bart pro xl bed probe bracket (Autodesk Fusion 360 design; units mm, degrees)
Autodesk Fusion 360 part; units mm, degrees
sketch "Sketch1" plane through (0, 0, 0) normal (0, 0, 1) x (1, 0, 0)
  circle A0 centre (25.3818, 25) radius 2
  line L0 (25.3818, 25) -> (25.3777, 25)
  line L1 (25.3777, 25) -> (48.3777, 25) construction
  circle A1 centre (48.3777, 25) radius 2
  line L2 (48.3777, 25) -> (48.3777, 26)
  line L3 (48.3777, 26) -> (48.3777, 32) construction
  line L4 (48.3777, 25) -> (54.3777, 25) construction
  line L5 (54.3777, 25) -> (54.3777, 0) construction
  line L6 (36.8777, 25) -> (36.8777, -5) construction
  line L7 (36.8777, 14.4744) -> (42.8777, 14.4744) construction
  line L8 (36.8777, 14.4744) -> (30.8777, 14.4744) construction
  line L9 (30.8777, 14.4744) -> (30.8777, 25) construction
  line L10 (42.8777, 14.4744) -> (42.8777, 25) construction
  line L11 (42.8777, 14.4744) -> (42.8777, 0) construction
  line L12 (30.8777, 14.4744) -> (30.8777, 0) construction
  line L13 (19.3777, 25) -> (19.3777, 24)
  line L14 (19.3777, 24) -> (19.3777, 0)
  arc A2 (25.3777, 31) -> (19.3777, 25) centre (25.3777, 25) ccw
  arc A3 (54.3777, 25) -> (48.3574, 31) centre (48.3777, 25) ccw
  line L15 (25.3777, 31) -> (48.3574, 31)
  line L16 (54.3777, 25) -> (54.3777, 0)
  line L17 (54.3777, 0) -> (52.8895, 0)
  arc A4 (42.8777, 19.7372) -> (30.8777, 19.7372) centre (36.8777, 18.9484) ccw
  line L18 (30.8777, 19.7372) -> (30.8777, 0)
  line L19 (42.8777, 19.7372) -> (42.8777, 0)
  line L20 (54.3777, 0) -> (42.8777, 0) construction
  line L21 (36.8777, 0) -> (15, 0) construction
  line L22 (19.3777, 0) -> (30.8777, 0)
  line L23 (42.8777, 0) -> (54.3777, 0)
  dimension "d1" = 4
  dimension "d2" = 23
  dimension "d3" = 4
  dimension "d6" = 25
  dimension "d7" = 39.3777
  dimension "d8" = 6
  dimension "d9" = 6
  dimension "d10" = 6
  constraint horizontal L0
  constraint perpendicular L1 L2
  constraint perpendicular L5 L20
  constraint midpoint L1
  constraint perpendicular L6 L20
  constraint coincident L6
  constraint coincident L1
  constraint perpendicular L1 L9
  constraint perpendicular L7 L10
  constraint perpendicular L11 L20
  constraint coincident L20
  constraint perpendicular L12 L20
  constraint perpendicular L14 L20
  constraint tangent A3 L16
  constraint coincident A4
  constraint midpoint L10
  constraint midpoint L9
  constraint perpendicular L18 L22
  constraint perpendicular L19 L22
  constraint collinear L20 L21
  constraint collinear L22 L23
  measures "d1" diameter of A0
  measures "d3" diameter of A1
extrude "Extrude1" add sketch "Sketch1" along normal blind 5
sketch "Sketch2" plane through (0, 0, 0) normal (0, -1, 0) x (1, 0, 0)
  line L0 (19.3777, 0) -> (30.8777, 0)
  line L1 (30.8777, 0) -> (30.8777, 5)
  line L2 (30.8777, 5) -> (19.3777, 5)
  line L3 (19.3777, 5) -> (19.3777, 0)
  line L4 (30.8777, 20) -> (19.3777, 20)
  line L5 (19.3777, 20) -> (19.3777, 0)
  line L6 (30.8777, 0) -> (30.8777, 20)
  dimension "d17" = 20
  constraint horizontal L4
  constraint vertical L5
  constraint perpendicular L4 L6
extrude "Extrude3" add sketch "Sketch2" against normal blind 5 contours L2 L4 L5 L6
sketch "Sketch4" plane through (0, 0, 0) normal (0, -1, 0) x (1, 0, 0)
  line L0 (42.8777, 0) -> (54.3777, 0)
  line L1 (54.3777, 0) -> (54.3777, 5)
  line L2 (54.3777, 5) -> (42.8777, 5)
  line L3 (42.8777, 5) -> (42.8777, 0)
  line L4 (42.8777, 0) -> (42.8777, 20)
  line L5 (54.3777, 0) -> (54.3777, 20)
  line L6 (42.8777, 20) -> (54.3777, 20)
  dimension "d20" = 20
  dimension "d21" = 20
  constraint perpendicular L4 L6
extrude "Extrude4" add sketch "Sketch4" against normal blind 5 contours L2 L4 L5 L6
sketch "Sketch5" plane through (0, 0, 0) normal (0, 1, 0) x (1, 0, 0)
  line L0 (42.8777, -20) -> (54.3777, -20)
  line L1 (37, -20) -> (37, 10) construction
  line L2 (48.3574, -5) -> (25.3777, -5)
  line L3 (42.8777, -5) -> (30.8777, -5)
  line L4 (39.9943, -5) -> (39.9943, -13) construction
  line L5 (39.9943, -13) -> (34, -13) construction
  line L6 (34, -13) -> (34, -19) construction
  circle A0 centre (36.9971, -13) radius 5.95 construction
  dimension "d24" = 8
  dimension "d25" = 6
  dimension "d26" = 11.9
  constraint perpendicular L0 L1
  constraint coincident L2
  constraint perpendicular L1 L5
  constraint midpoint L5
  measures "d26" diameter of A0
sketch "Sketch6" plane through (0, 0, 5) normal (0, 0, 1) x (-1, 0, 0)
  circle A0 centre (-48.3777, -25) radius 2
  circle A1 centre (-25.3818, -25) radius 2
  line L0 (-42.8777, -5) -> (-54.3777, -5)
  line L1 (-54.3777, -5) -> (-54.3777, -25)
  arc A2 (-54.3777, -25) -> (-48.3574, -31) centre (-48.3777, -25) ccw
  line L2 (-48.3574, -31) -> (-25.3777, -31)
  arc A3 (-25.3777, -31) -> (-19.3777, -25) centre (-25.3777, -25) ccw
  line L3 (-19.3777, -25) -> (-19.3777, -5)
  line L4 (-19.3777, -5) -> (-30.8777, -5)
  line L5 (-30.8777, -5) -> (-30.8777, -19.7372)
  arc A4 (-42.8777, -19.7372) -> (-30.8777, -19.7372) centre (-36.8777, -18.9484) ccw
  line L6 (-42.8777, -19.7372) -> (-42.8777, -5)
  line L7 (-28.0277, -26.53) -> (-25.3777, -28.06)
  line L8 (-25.3777, -28.06) -> (-22.7277, -26.53)
  line L9 (-22.7277, -26.53) -> (-22.7277, -23.47)
  line L10 (-22.7277, -23.47) -> (-25.3777, -21.94)
  line L11 (-25.3777, -21.94) -> (-28.0277, -23.47)
  line L12 (-28.0277, -23.47) -> (-28.0277, -26.53)
extrude "Extrude5" cut sketch "Sketch6" against normal blind 2.5 contours L7 L8 L9 L10 L11 L12
sketch "Sketch7" plane through (0, 0, 5) normal (0, 0, 1) x (-1, 0, 0)
  line L0 (-25.3777, -28.06) -> (-28.0277, -26.53)
  line L1 (-28.0277, -26.53) -> (-28.0277, -23.47)
  line L2 (-28.0277, -23.47) -> (-25.3777, -21.94)
  line L3 (-25.3777, -21.94) -> (-22.7277, -23.47)
  line L4 (-22.7277, -23.47) -> (-22.7277, -26.53)
  line L5 (-22.7277, -26.53) -> (-25.3777, -28.06)
  circle A0 centre (-48.3777, -25) radius 2
  line L6 (-42.8777, -5) -> (-54.3777, -5)
  line L7 (-54.3777, -5) -> (-54.3777, -25)
  arc A1 (-54.3777, -25) -> (-48.3574, -31) centre (-48.3777, -25) ccw
  line L8 (-48.3574, -31) -> (-25.3777, -31)
  arc A2 (-25.3777, -31) -> (-19.3777, -25) centre (-25.3777, -25) ccw
  line L9 (-19.3777, -25) -> (-19.3777, -5)
  line L10 (-19.3777, -5) -> (-30.8777, -5)
  line L11 (-30.8777, -5) -> (-30.8777, -19.7372)
  arc A3 (-42.8777, -19.7372) -> (-30.8777, -19.7372) centre (-36.8777, -18.9484) ccw
  line L12 (-42.8777, -19.7372) -> (-42.8777, -5)
  line L13 (-51.0277, -26.53) -> (-48.3777, -28.06)
  line L14 (-48.3777, -28.06) -> (-45.7277, -26.53)
  line L15 (-45.7277, -26.53) -> (-45.7277, -23.47)
  line L16 (-45.7277, -23.47) -> (-48.3777, -21.94)
  line L17 (-48.3777, -21.94) -> (-51.0277, -23.47)
  line L18 (-51.0277, -23.47) -> (-51.0277, -26.53)
extrude "Extrude6" cut sketch "Sketch7" against normal blind 2.5 contours L13 L14 L15 L16 L17 L18
